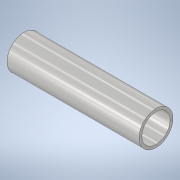
# Autodesk Inventor part: MC18_Rohr
Saved by Autodesk Inventor 2021 (Build 250183000, 183)
## iProperties
Created: 2020-04-27
Part Number: MC18_Rohr
Material: Aluminium 6061
Document SubType Name: Modeling
Designer: kaebi
Density: 2.7 g/cm^3
Appearance: Aluminium - dunkel
Description: Ausgaberohr
Stock Number: BEF 013 A
Mass: 14.6956 g
Surface Area: 74.1259 cm^2
Volume: 5.44281 cm^3
Author: kaebi
Autodesk Inventor part; units mm, degrees
ref_plane "YZ Plane" through (0, 0, 0) normal (1, 0, 0) x (0, 1, 0)
ref_plane "XZ Plane" through (0, 0, 0) normal (0, 1, 0) x (-1, 0, 0)
ref_plane "XY Plane" through (0, 0, 0) normal (0, 0, 1) x (1, 0, 0)
sketch "Skizze1" plane through (0, 0, 0) normal (1, 0, 0) x (0, 1, 0)
  circle A0 centre (0, 0) radius 7.5
  circle A1 centre (0, 0) radius 9
  dimension "d0" = 15
  dimension "d1" = 18
  constraints: 2 centre point, 1 coincident, 1 concentric
  measures "d0" diameter of A0
  measures "d1" diameter of A1
extrude "Extrusion1" add sketch "Skizze1" against normal blind 70
